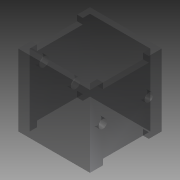
# Autodesk Inventor part: 13_0204_041
Saved by Autodesk Inventor 2012 SP1 (Build 160190100, 190)
## iProperties
Created: 2013-04-08
Part Number: 13_0204_041
Material: Default
Document SubType Name: Modeling
Designer: vogel
Density: 1 g/cm^3
Author: vogel
Autodesk Inventor part; units mm, degrees
ref_plane "YZ Plane" through (0, 0, 0) normal (1, 0, 0) x (0, 1, 0)
ref_plane "XZ Plane" through (0, 0, 0) normal (0, 1, 0) x (-1, 0, 0)
sketch "Skizze1" plane through (0, 0, 0) normal (0, 0, 1) x (1, 0, 0)
  line L0 (-12.5, 12.5) -> (12.5, 12.5)
  line L1 (12.5, 12.5) -> (12.5, -12.5)
  line L2 (12.5, -12.5) -> (-12.5, -12.5)
  line L3 (-12.5, -12.5) -> (-12.5, 12.5)
  line L4 (-17.5, 0) -> (17.5, 0) projected
  line L5 (0, -17.5) -> (0, 17.5) projected
  line L6 (10.5, 10.5) -> (-10.5, 10.5)
  line L7 (-10.5, 10.5) -> (-10.5, -10.5)
  line L8 (-10.5, -10.5) -> (10.5, -10.5)
  line L9 (10.5, -10.5) -> (10.5, 10.5)
  point P0 (0, 0)
  dimension "d0" = 25
  dimension "d1" = 25
  dimension "d2" = 2
  constraints: 16 end point, 4 parallel, 2 perpendicular, 1 horizontal, 5 other
  measures "d0" distance of L2.end L0.start
  measures "d1" distance of L0.start L0.end
  measures "d2" distance between parallel lines of L0 L6
extrude "Extrusion1" add sketch "Skizze1" along normal blind 25 contours L0 L5 L6 L7 L4 L3 | L0 L1 L4 L9 L6 L5 | L4 L7 L8 L5 L2 L3 | L1 L2 L5 L8 L9 L4
sketch "Skizze4" plane through (12.5, -12.5, 0) normal (1, 0, 0) x (0, 0, -1)
  line L0 (-25, 25) -> (-25, 0) projected
  line L1 (0, -5) -> (0, 30) projected
  line L2 (5, 12.5) -> (-30, 12.5) projected
  line L3 (-25, 20.5) -> (-23, 20.5)
  line L4 (-23, 20.5) -> (-23, 4.5)
  line L5 (-23, 4.5) -> (-25, 4.5)
  line L6 (-25, 4.5) -> (-25, 20.5)
  line L7 (0, 20.5) -> (-2, 20.5)
  line L8 (-2, 20.5) -> (-2, 4.5)
  line L9 (-2, 4.5) -> (0, 4.5)
  line L10 (0, 4.5) -> (0, 20.5)
  point P0 (0, 12.5)
  dimension "d9" = 16
  dimension "d10" = 2
  dimension "d11" = 2
  constraints: 16 end point, 4 parallel, 2 collinear, 2 horizontal, 2 perpendicular, 2 point on line, 1 other
  measures "d9" distance of L3.end L4.end
  measures "d10" distance of L3.start L3.end
  measures "d11" distance of L7.start L7.end
extrude "Extrusion3" cut sketch "Skizze4" against normal through all
ref_plane "Arbeitsebene2" through (0, 0, 12.5) normal (0, 0, -1) x (-1, 0, 0)
sketch "Skizze5" plane through (12.5, 12.5, 25) normal (1, 0, 0) x (0, 0, -1)
  line L0 (25, 0) -> (0, 0) projected
  line L1 (25, -25) -> (0, -25) projected
  line L2 (25, -30) -> (25, 5) projected
  line L3 (30, -12.5) -> (-5, -12.5) projected
  line L4 (12.5, -25) -> (12.5, 0)
  point P0 (25, -12.5)
  point P1 (12.5, -4.5)
  point P2 (12.5, -20.5)
  dimension "d15" = 16
  constraints: 2 end point, 2 midpoint, 2 point on line, 1 symmetric about line
  measures "d15" distance of point (12.5, -20.5) point (12.5, -4.5)
hole "Bohrung1" at (12.5, 8, 12.5) at (12.5, -8, 12.5) direction (-1, 0, 0) diameter 3 end up to surface
sketch "Skizze6" plane through (-12.5, -12.5, 0) normal (-1, 0, 0) x (0, 0, 1)
  point P0 (18.5, 7)
hole "Bohrung2" at (-12.5, -5.5, 18.5) direction (1, 0, 0) diameter 3.4 depth 2
sketch "Skizze7" plane through (-12.5, -12.5, 0) normal (-1, 0, 0) x (0, 0, 1)
  point P0 (6.5, 18)
hole "Bohrung4" at (-12.5, 5.5, 6.5) direction (1, 0, 0) diameter 3.4 depth 2
